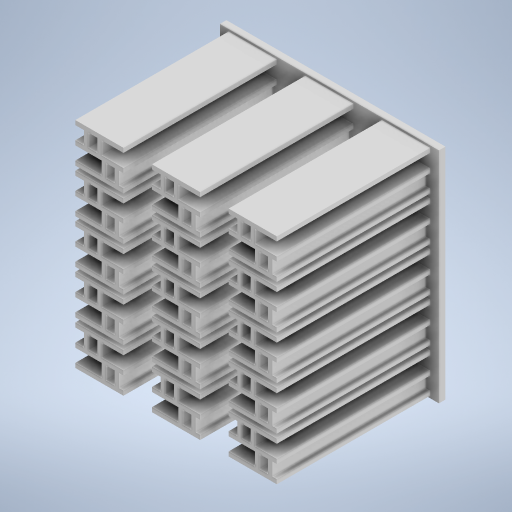
# Autodesk Inventor part: aletas
Saved by Autodesk Inventor 2023 (Build 270158000, 158)
## iProperties
Created: 2023-10-09
Part Number: aletas
Material: Generic
Document SubType Name: Modeling
Designer: Mauricio
Density: 1 g/cm^3
Appearance: Default
Author: Mauricio
Autodesk Inventor part; units mm, degrees
ref_plane "YZ Plane" through (0, 0, 0) normal (1, 0, 0) x (0, 1, 0)
ref_plane "XZ Plane" through (0, 0, 0) normal (0, 1, 0) x (-1, 0, 0)
ref_plane "XY Plane" through (0, 0, 0) normal (0, 0, 1) x (1, 0, 0)
sketch "Sketch1" plane through (0, 0, 0) normal (0, 0, 1) x (1, 0, 0)
  line L0 (0, 0) -> (22, 0)
  line L1 (22, 0) -> (22, -2)
  line L2 (0, -2) -> (0, 0)
  line L3 (6, -2) -> (6, -8)
  line L4 (4, -8) -> (4, -2)
  line L5 (12, -2) -> (12, -8)
  line L6 (10, -8) -> (10, -2)
  line L7 (22, -8) -> (22, -10)
  line L8 (0, -10) -> (0, -8)
  line L9 (14, -10) -> (14, -16)
  line L10 (12, -16) -> (12, -10)
  line L11 (20, -10) -> (20, -16)
  line L12 (18, -16) -> (18, -10)
  line L13 (0, -16) -> (0, -18)
  line L14 (0, -18) -> (22, -18)
  line L15 (22, -18) -> (22, -16)
  line L16 (12, -10) -> (0, -10)
  line L17 (12, -16) -> (0, -16)
  line L18 (22, -16) -> (20, -16)
  line L19 (18, -16) -> (14, -16)
  line L20 (22, -10) -> (20, -10)
  line L21 (18, -10) -> (14, -10)
  line L22 (12, -8) -> (22, -8)
  line L23 (0, -8) -> (4, -8)
  line L24 (6, -8) -> (10, -8)
  line L25 (22, -2) -> (12, -2)
  line L26 (10, -2) -> (6, -2)
  line L27 (4, -2) -> (0, -2)
  point P0 (0, -1)
  point P1 (13, -10)
  point P2 (19, -10)
  point P3 (0, -9)
  point P4 (16, -10)
  point P5 (8, -2)
  point P6 (21, -10)
  dimension "d1" = 22
  dimension "d2" = 2
  dimension "d3" = 2
  dimension "d4" = 4
  dimension "d5" = 4
  dimension "d8" = 2
  dimension "d9" = 2
  dimension "d10" = 2
  dimension "d13" = 4
  dimension "d15" = 2
  dimension "d16" = 2
  dimension "d17" = 2
  dimension "d18" = 2
  dimension "d20" = 2
  dimension "d21" = 2
  dimension "d22" = 2
  dimension "d23" = 6
  dimension "d24" = 6
  dimension "d25" = 6
  dimension "d26" = 2
  dimension "d27" = 6
  dimension "d28" = 6
  dimension "d29" = 1
  dimension "d30" = 2
  dimension "d31" = 2
  dimension "d32" = 1
  constraints: 56 end point, 22 parallel, 7 horizontal, 7 perpendicular, 5 midpoint, 4 vertical alignment
  measures "d1" distance from line of point (0, -1) L1
  measures "d2" distance between parallel lines of L3 L4
  measures "d3" distance between parallel lines of L5 L6
  measures "d4" distance between parallel lines of L2 L4
  measures "d5" distance between parallel lines of L6 L3
  measures "d8" distance between parallel lines of L7 L11
  measures "d9" distance between parallel lines of L11 L12
  measures "d10" distance between parallel lines of L10 L9
  measures "d13" distance between parallel lines of L12 L9
  measures "d15" distance between parallel lines of L0 L25
  measures "d16" distance between parallel lines of L0 L27
  measures "d17" distance between parallel lines of L0 L26
  measures "d18" distance between parallel lines of L16 L23
  measures "d20" distance between parallel lines of L16 L24
  measures "d21" distance from line of point (16, -10) L22
  measures "d22" distance between parallel lines of L20 L22
  measures "d23" distance between parallel lines of L22 L25
  measures "d24" distance from line of point (8, -2) L24
  measures "d25" distance between parallel lines of L17 L16
  measures "d26" distance between parallel lines of L17 L14
  measures "d27" distance between parallel lines of L21 L19
  measures "d28" distance from line of point (21, -10) L18
  measures "d29" distance from line of L11 point (19, -10)
  measures "d30" distance from line of L22 point (19, -10)
  measures "d31" distance from line of L22 point (13, -10)
  measures "d32" distance from line of L9 point (13, -10)
extrude "Extrusion1" add sketch "Sketch1" along normal blind 70
pattern_linear "Rectangular Pattern1" count 3 spacing 35 along (-1, 0, 0) count 5 spacing 20 along (0, 1, 0) of "Extrusion1"
sketch "Sketch4" plane through (22, 80, 0) normal (0, 0, -1) x (-1, 0, 0)
  line L0 (57, -16) -> (57, -18) projected
  line L1 (45, -16) -> (57, -16) projected
  line L2 (45, -10) -> (45, -16) projected
  line L3 (57, -10) -> (45, -10) projected
  line L4 (57, -8) -> (57, -10) projected
  line L5 (53, -8) -> (57, -8) projected
  line L6 (53, -2) -> (53, -8) projected
  line L7 (57, -2) -> (53, -2) projected
  line L8 (57, 0) -> (57, -2) projected
  line L9 (35, 0) -> (57, 0) projected
  line L10 (35, -2) -> (35, 0) projected
  line L11 (45, -2) -> (35, -2) projected
  line L12 (45, -8) -> (45, -2) projected
  line L13 (35, -8) -> (45, -8) projected
  line L14 (35, -10) -> (35, -8) projected
  line L15 (37, -10) -> (35, -10) projected
  line L16 (37, -16) -> (37, -10) projected
  line L17 (35, -16) -> (37, -16) projected
  line L18 (35, -18) -> (35, -16) projected
  line L19 (57, -18) -> (35, -18) projected
  line L20 (51, -2) -> (47, -2) projected
  line L21 (51, -8) -> (51, -2) projected
  line L22 (47, -8) -> (51, -8) projected
  line L23 (47, -2) -> (47, -8) projected
  line L24 (39, -16) -> (43, -16) projected
  line L25 (39, -10) -> (39, -16) projected
  line L26 (43, -10) -> (39, -10) projected
  line L27 (43, -16) -> (43, -10) projected
  line L28 (22, -56) -> (22, -58) projected
  line L29 (10, -56) -> (22, -56) projected
  line L30 (10, -50) -> (10, -56) projected
  line L31 (22, -50) -> (10, -50) projected
  line L32 (22, -48) -> (22, -50) projected
  line L33 (18, -48) -> (22, -48) projected
  line L34 (18, -42) -> (18, -48) projected
  line L35 (22, -42) -> (18, -42) projected
  line L36 (22, -40) -> (22, -42) projected
  line L37 (0, -40) -> (22, -40) projected
  line L38 (0, -42) -> (0, -40) projected
  line L39 (10, -42) -> (0, -42) projected
  line L40 (10, -48) -> (10, -42) projected
  line L41 (0, -48) -> (10, -48) projected
  line L42 (0, -50) -> (0, -48) projected
  line L43 (2, -50) -> (0, -50) projected
  line L44 (2, -56) -> (2, -50) projected
  line L45 (0, -56) -> (2, -56) projected
  line L46 (0, -58) -> (0, -56) projected
  line L47 (22, -58) -> (0, -58) projected
  line L48 (16, -42) -> (12, -42) projected
  line L49 (16, -48) -> (16, -42) projected
  line L50 (12, -48) -> (16, -48) projected
  line L51 (12, -42) -> (12, -48) projected
  line L52 (4, -56) -> (8, -56) projected
  line L53 (4, -50) -> (4, -56) projected
  line L54 (8, -50) -> (4, -50) projected
  line L55 (8, -56) -> (8, -50) projected
  line L56 (92, -56) -> (92, -58) projected
  line L57 (80, -56) -> (92, -56) projected
  line L58 (80, -50) -> (80, -56) projected
  line L59 (92, -50) -> (80, -50) projected
  line L60 (92, -48) -> (92, -50) projected
  line L61 (88, -48) -> (92, -48) projected
  line L62 (88, -42) -> (88, -48) projected
  line L63 (92, -42) -> (88, -42) projected
  line L64 (92, -40) -> (92, -42) projected
  line L65 (70, -40) -> (92, -40) projected
  line L66 (70, -42) -> (70, -40) projected
  line L67 (80, -42) -> (70, -42) projected
  line L68 (80, -48) -> (80, -42) projected
  line L69 (70, -48) -> (80, -48) projected
  line L70 (70, -50) -> (70, -48) projected
  line L71 (72, -50) -> (70, -50) projected
  line L72 (72, -56) -> (72, -50) projected
  line L73 (70, -56) -> (72, -56) projected
  line L74 (70, -58) -> (70, -56) projected
  line L75 (92, -58) -> (70, -58) projected
  line L76 (86, -42) -> (82, -42) projected
  line L77 (86, -48) -> (86, -42) projected
  line L78 (82, -48) -> (86, -48) projected
  line L79 (82, -42) -> (82, -48) projected
  line L80 (74, -56) -> (78, -56) projected
  line L81 (74, -50) -> (74, -56) projected
  line L82 (78, -50) -> (74, -50) projected
  line L83 (78, -56) -> (78, -50) projected
  line L84 (57, -96) -> (57, -98) projected
  line L85 (45, -96) -> (57, -96) projected
  line L86 (45, -90) -> (45, -96) projected
  line L87 (57, -90) -> (45, -90) projected
  line L88 (57, -88) -> (57, -90) projected
  line L89 (53, -88) -> (57, -88) projected
  line L90 (53, -82) -> (53, -88) projected
  line L91 (57, -82) -> (53, -82) projected
  line L92 (57, -80) -> (57, -82) projected
  line L93 (35, -80) -> (57, -80) projected
  line L94 (35, -82) -> (35, -80) projected
  line L95 (45, -82) -> (35, -82) projected
  line L96 (45, -88) -> (45, -82) projected
  line L97 (35, -88) -> (45, -88) projected
  line L98 (35, -90) -> (35, -88) projected
  line L99 (37, -90) -> (35, -90) projected
  line L100 (37, -96) -> (37, -90) projected
  line L101 (35, -96) -> (37, -96) projected
  line L102 (35, -98) -> (35, -96) projected
  line L103 (57, -98) -> (35, -98) projected
  line L104 (51, -82) -> (47, -82) projected
  line L105 (51, -88) -> (51, -82) projected
  line L106 (47, -88) -> (51, -88) projected
  line L107 (47, -82) -> (47, -88) projected
  line L108 (39, -96) -> (43, -96) projected
  line L109 (39, -90) -> (39, -96) projected
  line L110 (43, -90) -> (39, -90) projected
  line L111 (43, -96) -> (43, -90) projected
  line L112 (-4, 1) -> (96, 1)
  line L113 (96, 1) -> (96, -99)
  line L114 (96, -99) -> (-4, -99)
  line L115 (-4, -99) -> (-4, 1)
  line L116 (70, 0) -> (92, 0) projected
  line L117 (92, -98) -> (70, -98) projected
  line L118 (22, -88) -> (22, -90) projected
  line L119 (70, -2) -> (70, 0) projected
  line L120 (70, -20) -> (92, -20) projected
  line L121 (92, -18) -> (70, -18) projected
  point P0 (22, -80)
  point P1 (96, -49)
  point P2 (35, -89)
  point P3 (22, -89)
  point P4 (70, -1)
  point P5 (57, -1)
  dimension "d47" = 1
  dimension "d48" = 1
  dimension "d49" = 4
  dimension "d50" = 4
  dimension "d53" = 13
  dimension "d54" = 13
  dimension "d55" = 2
  constraints: 8 end point, 5 midpoint, 2 parallel, 1 horizontal, 1 perpendicular
  measures "d47" distance between parallel lines of L112 L116
  measures "d48" distance between parallel lines of L117 L114
  measures "d49" distance between parallel lines of L42 L115
  measures "d50" distance from line of point (96, -49) L60
  measures "d53" distance of point (35, -89) point (22, -89)
  measures "d54" distance of point (70, -1) point (57, -1)
  measures "d55" distance between parallel lines of L120 L121
extrude "Extrusion3" add sketch "Sketch4" along normal blind 3 contours L0 L19 L18 L17 L16 L15 L14 L13 L12 L11 L10 L9 L8 L7 L6 L5 L4 L3 L2 L1 | L21 L22 L23 L20 | L25 L26 L27 L24 | L28 L47 L46 L45 L44 L43 L42 L41 L40 L39 L38 L37 L36 L35 L34 L33 L32 L31 L30 L29 | L49 L50 L51 L48 | L53 L54 L55 L52 | L56 L75 L74 L73 L72 L71 L70 L69 L68 L67 L66 L65 L64 L63 L62 L61 L60 L59 L58 L57 | L77 L78 L79 L76 | L81 L82 L83 L80 | L84 L103 L102 L101 L100 L99 L98 L97 L96 L95 L94 L93 L92 L91 L90 L89 L88 L87 L86 L85 | L105 L106 L107 L104 | L109 L110 L111 L108 | L112 L113 L114 L115
equation "\"d1\" = 11 * d0"
equation "\"d2\" = d0"
equation "\"d3\" = d0"
equation "\"d4\" = 2 * d0"
equation "\"d5\" = d4"
equation "\"d8\" = d0"
equation "\"d9\" = d0"
equation "\"d10\" = d0"
equation "\"d13\" = 2 * d0"
equation "\"d15\" = d3"
equation "\"d16\" = d15"
equation "\"d17\" = d15"
equation "\"d18\" = d15"
equation "\"d20\" = d15"
equation "\"d21\" = d15"
equation "\"d22\" = d15"
equation "\"d23\" = 3 * d15"
equation "\"d24\" = 3 * d15"
equation "\"d25\" = 3 * d15"
equation "\"d26\" = d15"
equation "\"d27\" = 3 * d15"
equation "\"d28\" = 3 * d15"
equation "\"d29\" = 0.5 * d15"
equation "\"d30\" = d15"
equation "\"d31\" = d15"
equation "\"d32\" = 0.5 * d15"
equation "\"d33\" = 35 * d30"
equation "\"d7\" = d0"
equation "\"d14\" = d7"
equation "\"d0\" = 2"
body "Solid1"
